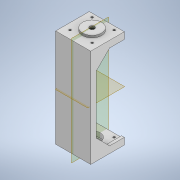
# Autodesk Inventor part: stepperMotorLink
Saved by Autodesk Inventor 2021 (Build 250183000, 183)
## iProperties
Created: 2021-03-14
Part Number: stepperMotorLink
Material: Generic
Document SubType Name: Modeling
Designer: awitc
Density: 1 g/cm^3
Appearance: Default
Author: awitc
Autodesk Inventor part; units mm, degrees
ref_plane "YZ Plane" through (0, 0, 0) normal (1, 0, 0) x (0, 1, 0)
ref_plane "XY Plane" through (0, 0, 0) normal (0, 0, 1) x (1, 0, 0)
sketch "Sketch1" plane through (0, 0, 0) normal (0, 1, 0) x (-1, 0, 0)
  line L0 (0, 0) -> (42, 0)
  line L1 (42, 0) -> (42, -42)
  line L2 (42, -42) -> (0, -42)
  line L3 (0, -42) -> (0, 0)
  line L4 (0, 0) -> (42, 0)
  line L5 (42, 0) -> (42, -42)
  line L6 (42, -42) -> (0, -42)
  line L7 (0, -42) -> (0, 0)
  line L8 (42, -21) -> (42, -5.25)
  circle A0 centre (36.75, -5.25) radius 1.5
  circle A1 centre (36.75, -36.75) radius 1.5
  circle A2 centre (5.25, -36.75) radius 1.5
  circle A3 centre (5.25, -5.25) radius 1.5
  dimension "d0" = 42
  dimension "d1" = 42
  dimension "d2" = 3
  dimension "d3" = 3
  dimension "d4" = 3
  dimension "d5" = 3
  constraints: 18 end point, 4 centre point, 4 parallel, 2 horizontal, 2 perpendicular, 1 midpoint, 1 point on line
  measures "d0" distance of L1.end L2.end
  measures "d1" distance of L0.end L1.end
  measures "d2" diameter of A0
  measures "d3" diameter of A1
  measures "d4" diameter of A2
  measures "d5" diameter of A3
extrude "Extrusion1" add sketch "Sketch1" along normal blind 5 and the other way blind 2.5
sketch "Sketch2" plane through (0, 5, 0) normal (0, 1, 0) x (1, 0, 0)
  circle A0 centre (-21, 21) radius 11.5
  point P0 (0, 0)
  point P1 (-42, 0)
  dimension "d9" = 23
  constraints: 1 centre point
  measures "d9" diameter of A0
extrude "Extrusion2" cut sketch "Sketch2" against normal up to surface (7.5 mm away)
sketch "Sketch3" plane through (0, 5, 0) normal (0, 1, 0) x (1, 0, 0)
  circle A0 centre (-21, 21) radius 11.5 projected
  circle A1 centre (-21, 21) radius 13.5
  circle A2 centre (-21, 21) radius 3.5
  point P0 (0, 0)
  dimension "d12" = 27
  dimension "d13" = 7
  constraints: 2 centre point, 2 coincident
  measures "d12" diameter of A1
  measures "d13" diameter of A2
extrude "Extrusion3" add sketch "Sketch3" along normal blind 3 contours A0 | A1
sketch "Sketch4" plane through (-42, -2.5, 0) normal (0, 0, 1) x (1, 0, 0)
  line L0 (42, 7.5) -> (42, 2.5) projected
  line L1 (42, 7.5) -> (0.1256, 7.5)
  line L2 (42, -112.5) -> (42, 7.5)
  line L3 (42, -112.5) -> (42, -122.5)
  line L4 (42, -132.5) -> (42, -122.5)
  line L5 (0, 0) -> (0, 7.5) projected
  line L6 (42, -132.5) -> (0, -132.5)
  line L7 (0, -132.5) -> (0, 7.5)
  line L8 (0, 7.5) -> (42, 7.5)
  line L9 (42, 7.5) -> (42, -132.5)
  point P0 (0.1256, 7.5)
  dimension "d20" = 10
  constraints: 16 end point, 2 horizontal, 2 parallel, 1 perpendicular
  measures "d20" distance of L3.start L3.end
extrude "Extrusion4" add sketch "Sketch4" along normal blind 6
ref_plane "Work Plane1" through (0, -62.5, 0) normal (0, 1, 0) x (-1, 0, 0)
ref_plane "Work Plane3" through (0, -65, 0) normal (0, 1, 0) x (1, 0, 0)
mirror "Mirror5" about plane through (0, -65, 0) normal (0, 1, 0) of "Extrusion1", "Extrusion3", "Extrusion2"
sketch "Sketch8" plane through (0, -2.5, -42) normal (1, 0, 0) x (0, 0, -1)
  line L0 (0, 7.5) -> (0, 0) projected
  line L1 (-48, -132.5) -> (-48, 7.5) projected
  line L2 (0, 7.5) -> (-48, 7.5)
  line L3 (-48, 7.5) -> (-48, -132.5)
  line L4 (-48, -132.5) -> (0, -132.5)
  line L5 (0, -132.5) -> (0, 7.5)
  line L6 (0, 0) -> (-42, 0) projected
  line L7 (-21.0744, 0) -> (-42, -20.9256)
  line L8 (-42, -125) -> (-42, 2.5) projected
  line L9 (-21.0744, 0) -> (8.5189, 0) construction
  line L10 (0, 0) -> (-42, 0)
  line L11 (-42, -20.9256) -> (-42, 2.5)
  line L12 (0, 7.5) -> (0, 0)
  line L13 (-21.0744, 0) -> (0, 0)
  line L14 (-42, -20.9256) -> (-42, -132.5)
  line L15 (0, -132.5) -> (-48, -132.5) projected
  line L16 (0, 0) -> (0, -2)
  line L17 (0, -2) -> (-21.0744, -2)
  line L18 (-21.0744, -2) -> (-21.0744, 0)
  line L19 (-21.0744, -2) -> (-42, -23)
  line L20 (-42, -23) -> (-40, -23)
  line L21 (-40.0407, -21.0337) -> (-40.0407, -130.0337)
  line L22 (-40.0407, -130.0337) -> (-40.0407, -132.5)
  dimension "d64" = 135
  dimension "d67" = 2
  constraints: 36 end point, 6 perpendicular, 6 point on line, 4 horizontal, 2 collinear, 2 parallel, 1 equal length, 1 vertical, 2 other
  measures "d64" angle of L7 L9
  measures "d67" distance of L0.end L16.end
extrude "Extrusion8" add sketch "Sketch8" along normal blind 4 contours L0 L6 L8 L14 L4 L1 L2 | L5 L17 L18 L6 | L7 L8 L6 | L18 L19 L8 L7 | L14 L8 L20 L21 L22 L4 | L21 L20 L19
mirror "Mirror6" about plane through (0, -65, 0) normal (0, 1, 0) of "Extrusion8"
ref_plane "Work Plane4" through (-21, -2.5, -42) normal (-1, 0, 0) x (0, 0, 1)
mirror "Mirror7" about plane through (-21, -2.5, -42) normal (-1, 0, 0) of "Extrusion8", "Mirror6"
sketch "Sketch9" plane through (0, -4.5, -42) normal (0, 0, -1) x (-1, 0, 0)
  line L0 (-4, 9.5) -> (-4, -130.5) projected
  line L1 (-4, 9.5) -> (-0.25, 9.5)
  line L2 (-0.25, 9.5) -> (-0.25, 5.75)
  line L3 (-0.25, 5.75) -> (-4, 5.75)
  line L4 (-4, 5.75) -> (-4, 9.5)
  line L5 (-4, -130.5) -> (46, -130.5) projected
  line L6 (46, -130.5) -> (42.25, -130.5)
  line L7 (42.25, -130.5) -> (42.25, -126.75)
  line L8 (42.25, -126.75) -> (46, -126.75)
  line L9 (46, -126.75) -> (46, -130.5)
  circle A0 centre (-0.25, 5.75) radius 1.5
  circle A1 centre (42.25, -126.75) radius 1.5
  circle A2 centre (42.25, 5.75) radius 1.5
  circle A3 centre (-0.25, -126.75) radius 1.5
  point P0 (0, 4.5)
  dimension "d71" = 3.75
  dimension "d72" = 3.75
  dimension "d73" = 3.75
  dimension "d74" = 3.75
  dimension "d75" = 3
  dimension "d76" = 3
  dimension "d77" = 3
  dimension "d78" = 3
  constraints: 16 end point, 4 centre point, 4 parallel, 2 coincident, 2 horizontal, 2 perpendicular
  measures "d71" distance of L2.end L3.end
  measures "d72" distance of L1.end L2.end
  measures "d73" distance of L7.end L8.end
  measures "d74" distance of L6.end L7.end
  measures "d75" diameter of A0
  measures "d76" diameter of A1
  measures "d77" diameter of A2
  measures "d78" diameter of A3
extrude "Extrusion9" cut sketch "Sketch9" against normal blind 15 contours A0 L2 L3 | L3 L2 A0 | A1 L8 L7 | L7 L8 A1 | A2 | A3
thread "Thread5" size "M3x0.5" class "6H" standard "ANSI Metric M Profile" full length
thread "Thread6" size "M3x0.5" class "6H" standard "ANSI Metric M Profile" full length
thread "Thread7" size "M3x0.5" class "6H" standard "ANSI Metric M Profile" full length
thread "Thread8" size "M3x0.5" class "6H" standard "ANSI Metric M Profile" full length
thread "Thread9" size "M3x0.5" class "6H" standard "ANSI Metric M Profile" full length
thread "Thread10" size "M3x0.5" class "6H" standard "ANSI Metric M Profile" full length
thread "Thread11" size "M3x0.5" class "6H" standard "ANSI Metric M Profile" full length
thread "Thread12" size "M3x0.5" class "6H" standard "ANSI Metric M Profile" full length
thread "Thread13" size "M3x0.5" class "6H" standard "ANSI Metric M Profile" full length
thread "Thread14" size "M3x0.5" class "6H" standard "ANSI Metric M Profile" full length
thread "Thread15" size "M3x0.5" class "6H" standard "ANSI Metric M Profile" full length
thread "Thread16" size "M3x0.5" class "6H" standard "ANSI Metric M Profile" full length
fillet "Fillet1" radius 1 1 edges at (-32.5, 5, -21)
fillet "Fillet2" radius 1 1 edges at (-32.5, -135, -21)
body "Solid1"
